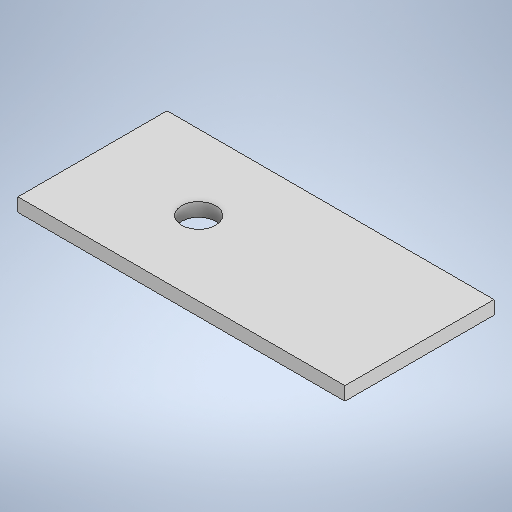
# Autodesk Inventor part: fire wall spacer
Saved by Autodesk Inventor 2025.2 (Build 292293000, 293)
## iProperties
Created: 2025-02-05
Part Number: fire wall spacer
Material: Generic
Document SubType Name: Modeling
Designer: 5013908
Density: 1 g/cm^3
Appearance: Default
Author: 5013908
Autodesk Inventor part; units mm, degrees
ref_plane "YZ Plane" through (0, 0, 0) normal (1, 0, 0) x (0, 1, 0)
ref_plane "XZ Plane" through (0, 0, 0) normal (0, 1, 0) x (-1, 0, 0)
ref_plane "XY Plane" through (0, 0, 0) normal (0, 0, 1) x (1, 0, 0)
sketch "Sketch1" plane through (0, 0, 0) normal (0, 1, 0) x (-1, 0, 0)
  line L0 (0, 0) -> (-76.7653, 0)
  line L1 (-76.7653, 0) -> (-76.7653, -35)
  line L2 (-76.7653, -35) -> (0, -35)
  line L3 (0, -35) -> (0, 0)
  circle A0 centre (-25, -17.4125) radius 4
  dimension "d0" = 35
  dimension "d1" = 76.7653
  dimension "d2" = 8
  dimension "d3" = 25
  dimension "d4" = 17.4125
  constraints: 8 end point, 2 parallel, 1 centre point, 1 horizontal, 1 perpendicular
  measures "d0" distance of L1.end L0.end
  measures "d1" distance of L1.end L2.end
  measures "d2" diameter of A0
  measures "d3" distance from line of A0.centre L3
  measures "d4" distance from line of A0.centre L0
extrude "Extrusion1" add sketch "Sketch1" along normal blind 3.175
body "Solid1"
